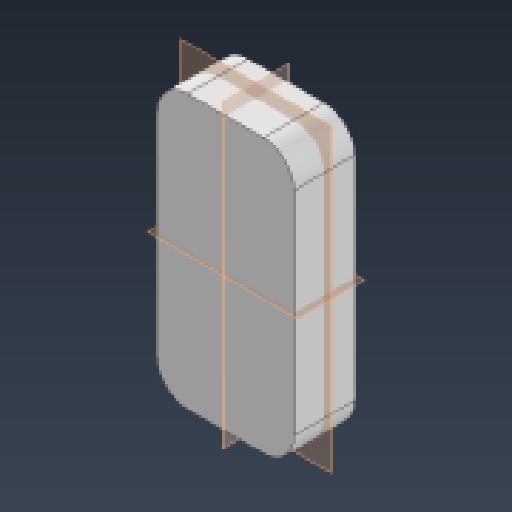
# Autodesk Inventor part: Основание
Saved by Autodesk Inventor 2023.2 (Build 272271030, 271C)
## iProperties
Created: 2026-01-03
Part Number: Основание
Material: Типовые
Document SubType Name: Modeling
Designer: Олег Коноваленко
Density: 1 g/cm^3
Appearance: По умолчанию
Author: Олег Коноваленко
Autodesk Inventor part; units mm, degrees
sketch "Эскиз1" plane through (0, 0, 0) normal (0, 0, 1) x (1, 0, 0)
  line L0 (-11.25, -22.5) -> (11.25, -22.5)
  line L1 (11.25, -22.5) -> (11.25, 22.5)
  line L2 (11.25, 22.5) -> (-11.25, 22.5)
  line L3 (-11.25, 22.5) -> (-11.25, -22.5)
  line L4 (-11.25, -22.5) -> (11.25, 22.5) construction
  line L5 (11.25, -22.5) -> (-11.25, 22.5) construction
  point P0 (0, 0)
  dimension "d0" = 45
  dimension "d1" = 22.5
  constraints: 12 end point, 2 midpoint, 2 parallel, 1 horizontal, 1 perpendicular
  measures "d0" distance of L0.end L1.end
  measures "d1" distance of L1.end L2.end
extrude "Выдавливание1" add sketch "Эскиз1" along normal mid plane 10.5
fillet "Сопряжение1" radius 5 4 edges at (11.25, 22.5, 0) (-11.25, 22.5, 0) (11.25, -22.5, 0) (-11.25, -22.5, 0)
sketch "Эскиз2" plane through (0, 0, 5.25) normal (0, 0, 1) x (1, 0, 0)
  circle A0 centre (6, -15) radius 1.5 projected
  circle A1 centre (-6, -15) radius 1.5 projected
  circle A2 centre (-6, 4) radius 1.5 projected
  circle A3 centre (6, 4) radius 1.5 projected
  point P0 (0, 0)
extrude "Выдавливание2" cut sketch "Эскиз2" against normal up to next
